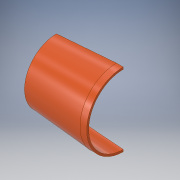
# Autodesk Inventor part: Blumentopf
Saved by Autodesk Inventor 2017 (Build 210142000, 142)
## iProperties
Part Number: Blumentopf
Material: Generisch
Document SubType Name: Modeling
Designer: OleSi
Density: 1 g/cm^3
Appearance: Glatt - hellorange
Author: OleSi
Autodesk Inventor part; units mm, degrees
ref_plane "YZ Plane" through (0, 0, 0) normal (1, 0, 0) x (0, 1, 0)
ref_plane "XZ Plane" through (0, 0, 0) normal (0, 1, 0) x (-1, 0, 0)
ref_plane "XY Plane" through (0, 0, 0) normal (0, 0, 1) x (1, 0, 0)
sketch "Skizze1" plane through (0, 0, 0) normal (1, 0, 0) x (0, 1, 0)
  circle A0 centre (0, 0) radius 55
  dimension "d0" = 110
  constraints: 1 centre point, 1 coincident
  measures "d0" diameter of A0
extrude "Extrusion1" add sketch "Skizze1" along normal blind 100
shell "Wandung1" thickness 10 removed faces 1 at (100, 13.749, -10.4033)
chamfer "Fase1" distance 7 distance2 90 1 edges at (100, -45, 0) measured on face at (100, -45.5, 0)
chamfer "Fase2" distance 7 distance2 90 1 edges at (0, -55, 0) measured on face at (0, -54.5, 0)
